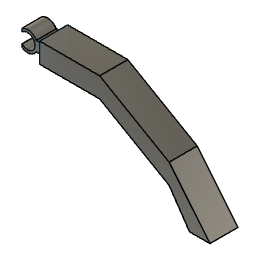
curved_singular_phalange v1 (Autodesk Fusion 360 design; units mm, degrees)
Autodesk Fusion 360 part; units mm, degrees
sketch "Sketch1" plane through (0, 0, 0) normal (0, 1, 0) x (1, 0, 0)
  line L0 (0, 0) -> (-30, 0)
  line L1 (-30, 0) -> (-30, -10)
  line L2 (-30, -10) -> (0, -10)
  line L3 (0, -10) -> (0, 0)
  line L4 (0, 0) -> (34.641, 20)
  line L5 (0, 0) -> (40, 0) construction
  line L6 (0, -10) -> (34.641, 10)
  line L7 (34.641, 10) -> (55, 35)
  line L8 (55, 35) -> (44.8205, 35)
  line L9 (44.8205, 35) -> (34.641, 20)
  dimension "d1" = 30
  dimension "d2" = 10
  dimension "d3" = 40
  dimension "d4" = 30
  constraint horizontal L0
  constraint vertical L1
  constraint horizontal L2
  constraint vertical L3
  constraint coincident L0.start L3.end
  constraint horizontal L5
  constraint parallel L4 L6
  constraint horizontal L8
  measures "d1" distance of L0.start L0.end
  measures "d2" distance of L0.start L2.end
  measures "d3" distance of L0.start L4.end
  measures "d4" angle of L4 L5
extrude "Extrude1" add sketch "Sketch1" along normal blind 14
sketch "Sketch2" plane through (-30, 0, 0) normal (-1, 0, 0) x (0, -1, 0)
  line L0 (0, 0) -> (0, 10)
  line L1 (0, 10) -> (-14, 10)
  line L2 (-14, 10) -> (-14, 0)
  line L3 (-14, 0) -> (0, 0)
sketch "Sketch3" plane through (-30, 0, 0) normal (-1, 0, 0) x (0, -1, 0)
  line L0 (-12, 7.5) -> (-2, 7.5)
  line L1 (-2, 7.5) -> (-2, 2.5)
  line L2 (-2, 2.5) -> (-12, 2.5)
  line L3 (-12, 2.5) -> (-12, 7.5)
  line L4 (-14, 10) -> (-14, 0)
  line L5 (0, 10) -> (-14, 10)
  dimension "d7" = 10
  dimension "d8" = 5
  dimension "d9" = 2
  dimension "d10" = 2.5
  constraint horizontal L0
  constraint vertical L1
  constraint horizontal L2
  constraint vertical L3
  measures "d7" distance of L0.start L0.end
  measures "d8" distance of L0.start L2.end
  measures "d9" distance of L3 L4
  measures "d10" distance of L0 L5
extrude "Extrude2" add sketch "Sketch3" along normal blind 5
cylinder "CylinderPrimitive1" add diameter 10 height -10 placed x (1, 0, 0) y (0, 0, -1) z (0, 1, 0) at (-37.9928, 12, 5)
sketch "Sketch5" plane through (0, 2, 0) normal (0, -1, 0) x (1, 0, 0)
  arc A0 (-33.6627, 7.5) -> (-33.6627, 2.5) centre (-37.9928, 5) ccw
  line L0 (-33.6627, 2.5) -> (-30, 2.5)
  line L1 (-30, 2.5) -> (-30, 7.5)
  line L2 (-30, 7.5) -> (-33.6627, 7.5)
  circle A1 centre (-37.9928, 5) radius 3.75
  dimension "d15" = 7.5
  constraint concentric A0 A1
  measures "d15" diameter of A1
extrude "Extrude3" cut sketch "Sketch5" against normal blind 35 contours A1
ref_plane "WorkPlane1" through (-45, 7, 5) normal (-1, 0, 0) x (0, -1, 0)
sketch "Sketch6" plane through (-45, 7, 5) normal (-1, 0, 0) x (0, 1, 0)
  line L0 (13.2157, -10.5168) -> (-13.0296, -10.5168)
  line L1 (-13.0296, -10.5168) -> (-13.0296, 7.5386)
  line L2 (-13.0296, 7.5386) -> (13.2157, 7.5386)
  line L3 (13.2157, 7.5386) -> (13.2157, -10.5168)
  constraint horizontal L0
  constraint vertical L1
  constraint horizontal L2
  constraint vertical L3
extrude "Extrude4" cut sketch "Sketch6" against normal blind 4.25
sketch "Sketch7" plane through (0, 2, 0) normal (0, -1, 0) x (1, 0, 0)
  line L0 (-40.75, 2.4583) -> (-40.75, 0.8289)
  arc A0 (-40.75, 0.8289) -> (-33.6627, 2.5) centre (-37.9928, 5) ccw
  line L1 (-33.6627, 2.5) -> (-30, 2.5)
  line L2 (-30, 2.5) -> (-30, 7.5)
  line L3 (-30, 7.5) -> (-33.6627, 7.5)
  arc A1 (-33.6627, 7.5) -> (-40.75, 9.1711) centre (-37.9928, 5) ccw
  line L4 (-40.75, 9.1711) -> (-40.75, 7.5417)
  arc A2 (-40.75, 2.4583) -> (-40.75, 7.5417) centre (-37.9928, 5) ccw
